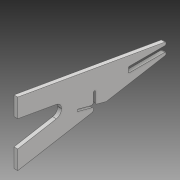
# Autodesk Inventor part: stand_insTop
Saved by Autodesk Inventor 2017 (Build 210142000, 142)
## iProperties
Created: 2019-02-02
Part Number: stand_insTop
Material: Generic
Document SubType Name: Modeling
Designer: ari
Density: 1 g/cm^3
Appearance: Default
Author: ari
Autodesk Inventor part; units mm, degrees
ref_plane "YZ Plane" through (0, 0, 0) normal (1, 0, 0) x (0, 1, 0)
ref_plane "XZ Plane" through (0, 0, 0) normal (0, 1, 0) x (-1, 0, 0)
ref_plane "XY Plane" through (0, 0, 0) normal (0, 0, 1) x (1, 0, 0)
sketch "Sketch1" plane through (0, 0, 0) normal (1, 0, 0) x (0, 1, 0)
  line L0 (0, 0) -> (237, -41.7895)
  line L1 (237, -41.7895) -> (237, -46.4413)
  line L2 (237, -60.0931) -> (141.6124, -76.9125)
  line L3 (0, -101.8825) -> (0, -71.8825)
  line L4 (0, -71.8825) -> (70, -59.5397)
  line L5 (70, -59.5397) -> (70, -42.3429)
  line L6 (70, -42.3429) -> (0, -30)
  line L7 (0, -30) -> (0, 0)
  line L8 (177, -50.9413) -> (70, -50.9413) construction
  line L9 (237, -46.4413) -> (177, -46.4413)
  line L10 (177, -46.4413) -> (177, -55.4413)
  line L11 (177, -55.4413) -> (237, -55.4413)
  line L12 (237, -55.4413) -> (237, -46.4413) construction
  line L13 (237, -46.4413) -> (237, -55.4413) construction
  line L14 (237, -55.4413) -> (237, -60.0931)
  line L15 (-47.4, 0) -> (284.4, 0) construction
  line L16 (124.05, -80.0092) -> (124.05, -72.2066)
  line L17 (121, -80.547) -> (121, -71.3894)
  arc A0 (124.05, -54.0092) -> (121, -54.0092) centre (122.525, -54.0092) ccw
  line L18 (122.525, -54.0092) -> (122.525, -21.6045) construction
  line L19 (121, -71.3894) -> (96.8519, -64.9189)
  line L20 (121, -74.547) -> (96.0625, -67.865)
  arc A1 (96.8519, -64.9189) -> (96.0625, -67.865) centre (96.4572, -66.392) ccw
  line L21 (121, -71.3894) -> (141.6124, -76.9125)
  line L22 (141.6124, -76.9125) -> (0, -101.8825)
  line L23 (124.05, -72.2066) -> (124.05, -54.0092)
  line L24 (121, -71.3894) -> (121, -54.0092)
  dimension "d2" = 9
  dimension "d3" = 60
  dimension "d4" = 177
  dimension "d5" = 30
  dimension "d7" = 10
  dimension "d9" = 15
  dimension "d10" = 101.8825
  dimension "d11" = 237
  dimension "d17" = 3.05
  dimension "d20" = 51
  dimension "d22" = 25
  dimension "d23" = 6
  dimension "d24" = 15
  dimension "d25" = 26
  dimension "d26" = 70
  constraints: 48 end point, 11 parallel, 8 vertical, 7 point on line, 6 tangent, 4 point on circle, 3 collinear, 2 centre point, 2 horizontal, 2 midpoint, 1 equal radius, 1 perpendicular, 2 other
  measures "d2" distance between parallel lines of L11 L9
  measures "d3" distance of L10.end L11.end
  measures "d4" distance between parallel lines of L7 L10
  measures "d5" distance of L6.end L0.start
  measures "d7" angle of L0 L15
  measures "d9" distance from line of L0 L9.end
  measures "d10" distance of L3.start L0.start
  measures "d11" horizontal distance of L0.end L0.start
  measures "d17" distance between parallel lines of L16 L17
  measures "d20" distance between parallel lines of L17 L5
  measures "d22" distance of L17.end L19.end
  measures "d23" distance of L17.start L20.start
  measures "d24" angle of L8 L19
  measures "d25" distance of L16.start L23.end
  measures "d26" distance between parallel lines of L3 L5
extrude "Extrusion1" add sketch "Sketch1" along normal blind 6 contours L0 L1 L9 L10 L11 L14 L2 L21 L23 A0 L24 L19 A1 L20 L17 L22 L3 L4 L5 L6 L7
fillet "Fillet1" radius 10 2 edges at (3, 70, -59.5397) (3, 70, -42.3429)
fillet "Fillet1" radius 1 2 edges at (3, 177, -55.4413) (3, 177, -46.4413)
fillet "Fillet1" radius 3 4 edges at (3, 124.05, -72.2066) (3, 121, -71.3894) (3, 121, -74.547) (3, 121, -80.547)
fillet "Fillet1" radius 2 4 edges at (3, 237, -60.0931) (3, 237, -55.4413) (3, 237, -46.4413) (3, 237, -41.7895)
equation "\"d17\" = d + u"
equation "\"d15\" = d23"
equation "\"d\" = 3"
equation "\"u\" = 0.05"
body "Solid1"
